90º rotrory adaper (Autodesk Fusion 360 design; units mm, degrees)
Autodesk Fusion 360 part; units mm, degrees
sketch "Sketch2" plane through (0, 0, 0) normal (0, 0, 1) x (1, 0, 0)
  line L0 (-6, 6) -> (6, 6)
  line L1 (6, 6) -> (6, -6)
  line L2 (6, -6) -> (-6, -6)
  line L3 (-6, -6) -> (-6, 6)
  line L4 (-6, 6) -> (6, -6) construction
  line L5 (6, 6) -> (-6, -6) construction
  dimension "d1" = 12
  dimension "d2" = 12
  constraint horizontal L0
  constraint perpendicular L0 L1
  constraint parallel L0 L2
  constraint parallel L1 L3
  constraint coincident L4 origin
  constraint coincident L5 origin
  measures "d1" distance of L0.start L0.end
  measures "d2" distance of L0 L2
extrude "Extrude1" add sketch "Sketch2" along normal blind 14 makes body 1
sketch "Sketch3" plane through (0, -6, 0) normal (0, -1, 0) x (1, 0, 0)
  line L0 (-6, 0) -> (6, 0)
  line L1 (6, 0) -> (6, 14)
  line L2 (6, 14) -> (-6, 14)
  line L3 (-6, 14) -> (-6, 0)
  line L4 (-6, 0) -> (6, 0)
  line L5 (6, 0) -> (6, -30.9661)
  line L6 (6, -30.9661) -> (-6, -30.9661)
  line L7 (-6, -30.9661) -> (-6, 0)
  line L8 (0, 0) -> (0, -30.9661) construction
  line L9 (13, -19.7077) -> (6.5, -8.4494)
  line L10 (6.5, -8.4494) -> (-6.5, -8.4494)
  line L11 (-6.5, -8.4494) -> (-13, -19.7077)
  line L12 (-13, -19.7077) -> (-6.5, -30.9661)
  line L13 (-6.5, -30.9661) -> (6.5, -30.9661)
  line L14 (6.5, -30.9661) -> (13, -19.7077)
  point P0 (0, -19.7077)
  dimension "d5" = 13
  constraint horizontal L4
  constraint vertical L5
  constraint horizontal L6
  constraint vertical L7
  constraint coincident L0.start L3.end
  constraint coincident L0.end L1.start
  constraint coincident L8.start origin
  constraint midpoint L6 L8.end
  constraint coincident L8 P0
  constraint horizontal L13
  constraint coincident L6 L12.end
  measures "d5" distance of L9.start L13.end
extrude "Extrude2" add sketch "Sketch3" along normal blind 17 separate body contours L5 L6 L7 L10 L13 | L7 L10 L11 L12 L13 | L5 L9 L10 L13 L14 makes body 2
extrude "Extrude3" add 1 faces at (2, -6, -23.4605) along direction (0, 1, 0) blind 12 on bodies 2 bodies 2
extrude "Extrude4" add 1 faces at (2, -2, 0) along direction (0, 0, -1) blind 10.3851 on bodies 1 bodies 1 2
